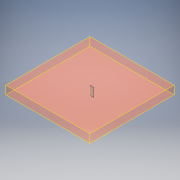
# Autodesk Inventor part: NACA63-015
Saved by Autodesk Inventor 2018 (Build 220112000, 112)
## iProperties
Created: 2019-05-16
Part Number: NACA63-015
Material: 一般
Document SubType Name: Modeling
Designer: Fluidlab
Density: 1 g/cm^3
Appearance: 既定
Author: Fluidlab
Autodesk Inventor part; units mm, degrees
ref_plane "YZ Plane" through (0, 0, 0) normal (1, 0, 0) x (0, 1, 0)
ref_plane "XZ Plane" through (0, 0, 0) normal (0, 1, 0) x (-1, 0, 0)
ref_plane "XY Plane" through (0, 0, 0) normal (0, 0, 1) x (1, 0, 0)
sketch "スケッチ1" plane through (0, 0, 0) normal (0, 0, 1) x (1, 0, 0)
  spline S0 degree 4 poles (1, 0.0003) (0.9688, 0.0049) (0.925, 0.0114) (0.8688, 0.0198) (0.8, 0.0299) (0.75, 0.0373) (0.7, 0.0448) (0.6501, 0.0518) (0.6001, 0.0584) (0.5501, 0.0641) (0.5001, 0.0688) (0.4501, 0.0724) (0.4, 0.0747) (0.35, 0.0753) (0.2998, 0.0742) (0.2503, 0.0713) (0.1996, 0.0664) (0.1564, 0.061) (0.1022, 0.051) (0.0783, 0.0447) (0.0531, 0.0381) (0.0285, 0.0278) (0.015, 0.021) (0.007, 0.0138) (0.0052, 0.0129) (-0.0034, 0) (0.0052, -0.0129) (0.007, -0.0138) (0.015, -0.021) (0.0285, -0.0278) (0.0531, -0.0381) (0.0783, -0.0447) (0.1022, -0.051) (0.1564, -0.061) (0.1996, -0.0664) (0.2503, -0.0713) (0.2998, -0.0742) (0.35, -0.0753) (0.4, -0.0747) (0.4501, -0.0724) (0.5001, -0.0688) (0.5501, -0.0641) (0.6001, -0.0584) (0.6501, -0.0518) (0.7, -0.0448) (0.75, -0.0373) (0.8, -0.0299) (0.8688, -0.0198) (0.925, -0.0114) (0.9688, -0.0049) (1, -0.0003) knots 0 0 0 0 0 0.057355 0.080296 0.103238 0.126177 0.149108 0.172027 0.194928 0.217807 0.240666 0.263507 0.286336 0.309162 0.331999 0.354861 0.377772 0.399068 0.418771 0.436942 0.45243 0.465861 0.476678 0.486208 0.495579 0.504421 0.513792 0.523322 0.534139 0.54757 0.563058 0.581229 0.600932 0.622228 0.645139 0.668001 0.690838 0.713664 0.736493 0.759334 0.782193 0.805072 0.827973 0.850892 0.873823 0.896762 0.919704 0.942645 1 1 1 1 1
  line L0 (1, 0.0003) -> (1, -0.0003)
  point P0 (0.95, 0.0077)
  point P1 (0.9, 0.0151)
  point P2 (0.85, 0.0225)
  point P3 (0.8, 0.0299)
  point P4 (0.75, 0.0373)
  point P5 (0.7, 0.0447)
  point P6 (0.65, 0.0517)
  point P7 (0.6, 0.0582)
  point P8 (0.55, 0.0639)
  point P9 (0.5, 0.0686)
  point P10 (0.45, 0.0722)
  point P11 (0.4, 0.0743)
  point P12 (0.35, 0.075)
  point P13 (0.3, 0.0738)
  point P14 (0.25, 0.0709)
  point P15 (0.2, 0.0662)
  point P16 (0.15, 0.0594)
  point P17 (0.1, 0.05)
  point P18 (0.075, 0.0438)
  point P19 (0.05, 0.0362)
  point P20 (0.025, 0.0258)
  point P21 (0.0125, 0.0184)
  point P22 (0.0075, 0.0145)
  point P23 (0.005, 0.012)
  point P24 (0, 0)
  point P25 (0.005, -0.012)
  point P26 (0.0075, -0.0145)
  point P27 (0.0125, -0.0184)
  point P28 (0.025, -0.0258)
  point P29 (0.05, -0.0362)
  point P30 (0.075, -0.0438)
  point P31 (0.1, -0.05)
  point P32 (0.15, -0.0594)
  point P33 (0.2, -0.0662)
  point P34 (0.25, -0.0709)
  point P35 (0.3, -0.0738)
  point P36 (0.35, -0.075)
  point P37 (0.4, -0.0743)
  point P38 (0.45, -0.0722)
  point P39 (0.5, -0.0686)
  point P40 (0.55, -0.0639)
  point P41 (0.6, -0.0582)
  point P42 (0.65, -0.0517)
  point P43 (0.7, -0.0447)
  point P44 (0.75, -0.0373)
  point P45 (0.8, -0.0299)
  point P46 (0.85, -0.0225)
  point P47 (0.9, -0.0151)
  point P48 (0.95, -0.0077)
  constraints: 2 end point, 1 vertical, 52 other
extrude "押し出し1" add sketch "スケッチ1" along normal blind 2
sketch "スケッチ2" plane through (0, 0, 2) normal (0, 0, 1) x (1, 0, 0)
  line L0 (-10, 10) -> (10, 10)
  line L1 (10, 10) -> (10, -10)
  line L2 (10, -10) -> (-10, -10)
  line L3 (-10, -10) -> (-10, 10)
  point P0 (0, 0)
  dimension "d2" = 20
  dimension "d3" = 20
  dimension "d5" = 10
  dimension "d12" = 10
  constraints: 8 end point, 2 parallel, 1 horizontal, 1 perpendicular
  measures "d2" distance of L0.end L1.end
  measures "d3" distance of L1.end L2.end
  measures "d5" distance from line of L0 point (0, 0)
  measures "d12" distance from line of L3 point (0, 0)
surface extrude "押し出しサーフェス1" sketch "スケッチ2" against normal blind 2 shown yes curves L0 L1 L2 L3
sketch "スケッチ3" plane through (-10, 10, 2) normal (0, 1, 0) x (1, 0, 0)
  line L0 (0, 0) -> (20, 0) projected
  line L1 (0, 2) -> (20, 2) projected
  point P0 (10, 2)
surface extrude "押し出しサーフェス2" sketch "スケッチ3" against normal up to surface (20 mm away) shown yes curves L1
sketch "スケッチ4" plane through (-10, 10, 2) normal (0, 1, 0) x (1, 0, 0)
  line L0 (0, 0) -> (20, 0) projected
  point P0 (10, 2)
surface extrude "押し出しサーフェス3" sketch "スケッチ4" against normal up to surface (20 mm away) shown yes curves L0
move or copy body "ボディを移動1" bodies to move or copy 1 copy no rotation origin (0, 0, 0) rotation axis (0, 0, 1) rotation angle -5
body "Srf1"
body "Srf2"
body "Srf3"
